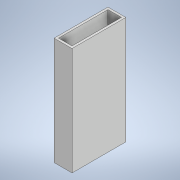
# Autodesk Inventor part: 2x4 StandIn- 2021
Saved by Autodesk Inventor 2021 (Build 250183000, 183)
## iProperties
Created: 2021-03-23
Part Number: 2x4 StandIn- 2021
Material: Generic
Document SubType Name: Modeling
Designer: con_c_000
Density: 1 g/cm^3
Appearance: Default
Author: con_c_000
Autodesk Inventor part; units mm, degrees
ref_plane "YZ Plane" through (0, 0, 0) normal (1, 0, 0) x (0, 1, 0)
ref_plane "XZ Plane" through (0, 0, 0) normal (0, 1, 0) x (-1, 0, 0)
ref_plane "XY Plane" through (0, 0, 0) normal (0, 0, 1) x (1, 0, 0)
sketch "Sketch1" plane through (0, 0, 0) normal (0, 1, 0) x (-1, 0, 0)
  line L0 (-12.7, 76.2) -> (12.7, 76.2)
  line L1 (12.7, 76.2) -> (12.7, 0)
  line L2 (12.7, 0) -> (-12.7, 0)
  line L3 (-12.7, 0) -> (-12.7, 76.2)
  line L4 (9.525, 73.025) -> (-9.525, 73.025)
  line L5 (-9.525, 73.025) -> (-9.525, 3.175)
  line L6 (-9.525, 3.175) -> (9.525, 3.175)
  line L7 (9.525, 3.175) -> (9.525, 73.025)
  point P0 (0, 0)
  dimension "d0" = 25.4
  dimension "d1" = 76.2
  dimension "d2" = 0
  dimension "d3" = 12.7
  dimension "d4" = 3.175
  constraints: 16 end point, 4 parallel, 2 perpendicular, 1 horizontal, 3 other
  measures "d0" distance of L1.end L2.end
  measures "d1" distance of L0.end L1.end
  measures "d2" distance from line of point (0, 0) L2
  measures "d3" distance from line of point (0, 0) L3
  measures "d4" distance between parallel lines of L0 L4
extrude "Extrusion1" add sketch "Sketch1" along normal mid plane 152.4
body "Solid1"
